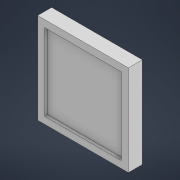
# Autodesk Inventor part: Clip_MarkerHolderV1
Saved by Autodesk Inventor 2022 (Build 260153000, 153)
## iProperties
Created: 2023-05-06
Part Number: Clip_MarkerHolderV1
Material: Generic
Document SubType Name: Modeling
Designer: Karl Spiteri
Density: 1 g/cm^3
Appearance: Default
Author: Karl Spiteri
Autodesk Inventor part; units mm, degrees
ref_plane "YZ Plane" through (0, 0, 0) normal (1, 0, 0) x (0, 1, 0)
ref_plane "XZ Plane" through (0, 0, 0) normal (0, 1, 0) x (-1, 0, 0)
ref_plane "XY Plane" through (0, 0, 0) normal (0, 0, 1) x (1, 0, 0)
sketch "Sketch5" plane through (0, 0, 0) normal (0, 0, 1) x (1, 0, 0)
  circle A0 centre (0, 0) radius 14.35
  circle A1 centre (0, 0) radius 16.85
  line L0 (32.5, 32.5) -> (-32.5, 32.5)
  line L1 (-32.5, 32.5) -> (-32.5, -32.5)
  line L2 (-32.5, -32.5) -> (32.5, -32.5)
  line L3 (32.5, -32.5) -> (32.5, 32.5)
  line L4 (-27.5, 27.5) -> (27.5, 27.5)
  line L5 (27.5, 27.5) -> (27.5, -27.5)
  line L6 (27.5, -27.5) -> (-27.5, -27.5)
  line L7 (-27.5, -27.5) -> (-27.5, 27.5)
  dimension "d36" = 28.7
  dimension "d37" = 33.7
  dimension "d38" = 65
  dimension "d39" = 65
  dimension "d40" = 55
  dimension "d41" = 55
  constraints: 16 end point, 4 parallel, 2 centre point, 2 coincident, 2 horizontal, 2 perpendicular
  measures "d36" diameter of A0
  measures "d37" diameter of A1
  measures "d38" distance of L2.end L1.end
  measures "d39" distance of L1.end L0.end
  measures "d40" distance of L5.end L6.end
  measures "d41" distance of L4.end L5.end
extrude "Extrusion7" add sketch "Sketch5" along normal blind 10 contours A0 | A1 | L3 L2 L1 L0 | L4 L5 L6 L7
sketch "Sketch6" plane through (0, 0, 0) normal (0, 0, -1) x (-1, 0, 0)
  circle A0 centre (0, 0) radius 14.35
  circle A1 centre (0, 0) radius 17.15
  line L0 (-27.5, 27.5) -> (27.5, 27.5)
  line L1 (27.5, 27.5) -> (27.5, -27.5)
  line L2 (27.5, -27.5) -> (-27.5, -27.5)
  line L3 (-27.5, -27.5) -> (-27.5, 27.5)
  dimension "d44" = 28.7
  dimension "d45" = 34.3
  dimension "d46" = 55
  dimension "d47" = 55
  constraints: 8 end point, 2 centre point, 2 coincident, 2 parallel, 1 horizontal, 1 perpendicular
  measures "d44" diameter of A0
  measures "d45" diameter of A1
  measures "d46" distance of L1.end L2.end
  measures "d47" distance of L0.end L1.end
extrude "Extrusion8" cut sketch "Sketch6" against normal blind 5 contours A1
sketch "Sketch7" plane through (0, 0, 10) normal (0, 0, 1) x (1, 0, 0)
  line L0 (-27.5, 27.5) -> (27.5, 27.5)
  line L1 (27.5, 27.5) -> (27.5, -27.5)
  line L2 (27.5, -27.5) -> (-27.5, -27.5)
  line L3 (-27.5, -27.5) -> (-27.5, 27.5)
  point P0 (0, 0)
  dimension "d50" = 55
  dimension "d51" = 55
  constraints: 8 end point, 2 parallel, 1 horizontal, 1 perpendicular
  measures "d50" distance of L1.end L2.end
  measures "d51" distance of L0.end L1.end
extrude "Extrusion9" cut sketch "Sketch7" against normal blind 2
body "Solid2"
